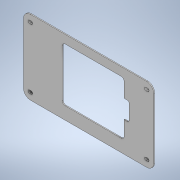
# Autodesk Inventor part: Navi base plate
Saved by Autodesk Inventor 2022 (Build 260153000, 153)
## iProperties
Created: 2021-09-22
Part Number: Navi base plate
Material: Generic
Document SubType Name: Modeling
Designer: Frank
Density: 1 g/cm^3
Appearance: Default
Author: Frank
Autodesk Inventor part; units mm, degrees
ref_plane "YZ Plane" through (0, 0, 0) normal (1, 0, 0) x (0, 1, 0)
ref_plane "XZ Plane" through (0, 0, 0) normal (0, 1, 0) x (-1, 0, 0)
ref_plane "XY Plane" through (0, 0, 0) normal (0, 0, 1) x (1, 0, 0)
sketch "Sketch1" plane through (0, 0, 0) normal (0, 0, 1) x (1, 0, 0)
  line L0 (-88.6, 55.18) -> (88.6, 55.18)
  line L1 (96.28, 47.5) -> (96.28, -47.5)
  line L2 (88.6, -55.18) -> (-88.6, -55.18)
  line L3 (-96.28, -47.5) -> (-96.28, 47.5)
  arc A0 (-96.28, -47.5) -> (-88.6, -55.18) centre (-88.6, -47.5) ccw
  arc A1 (88.6, -55.18) -> (96.28, -47.5) centre (88.6, -47.5) ccw
  arc A2 (96.28, 47.5) -> (88.6, 55.18) centre (88.6, 47.5) ccw
  arc A3 (-88.6, 55.18) -> (-96.28, 47.5) centre (-88.6, 47.5) ccw
  line L4 (85, 52.5) -> (-85, 52.5)
  line L5 (-85, 52.5) -> (-85, -52.5)
  line L6 (-85, -52.5) -> (85, -52.5)
  line L7 (85, -52.5) -> (85, 52.5)
  line L8 (85, 52.5) -> (-85, -52.5) construction
  line L9 (-85, 52.5) -> (85, -52.5) construction
  line L10 (0, -55.18) -> (0, 55.18) construction
  line L11 (-96.28, 0) -> (96.28, 0) construction
  line L12 (88.6, -47.5) -> (-88.6, -47.5) construction
  line L13 (-88.6, -47.5) -> (-88.6, 47.5) construction
  line L14 (-88.6, 47.5) -> (88.6, 47.5) construction
  line L15 (88.6, 47.5) -> (88.6, -47.5) construction
  line L16 (-92.28, -50) -> (-92.28, 50)
  line L17 (-92.28, -50) -> (-85, -50)
  line L18 (-92.28, 50) -> (-85, 50)
  line L19 (64.35, -31.825) -> (64.35, 33.825) construction
  line L20 (64.35, 33.825) -> (-61.85, 33.825) construction
  line L21 (-61.85, 33.825) -> (-61.85, -31.825) construction
  line L22 (-61.85, -31.825) -> (64.35, -31.825) construction
  line L23 (-61.85, 33.825) -> (64.35, -31.825) construction
  line L24 (-61.85, -31.825) -> (64.35, 33.825) construction
  line L25 (1.25, 0) -> (1.25, 1) construction
  line L26 (1.25, 1) -> (0, 1) construction
  line L27 (63.525, -31.825) -> (65.175, -31.825) construction
  line L28 (63.525, -30.175) -> (65.175, -30.175)
  line L29 (65.175, -33.475) -> (63.525, -33.475)
  arc A4 (63.525, -30.175) -> (63.525, -33.475) centre (63.525, -31.825) ccw
  arc A5 (65.175, -33.475) -> (65.175, -30.175) centre (65.175, -31.825) ccw
  line L30 (63.525, 33.825) -> (65.175, 33.825) construction
  line L31 (63.525, 35.475) -> (65.175, 35.475)
  line L32 (65.175, 32.175) -> (63.525, 32.175)
  arc A6 (63.525, 35.475) -> (63.525, 32.175) centre (63.525, 33.825) ccw
  arc A7 (65.175, 32.175) -> (65.175, 35.475) centre (65.175, 33.825) ccw
  line L33 (-61.025, 33.825) -> (-62.675, 33.825) construction
  line L34 (-61.025, 35.475) -> (-62.675, 35.475)
  line L35 (-62.675, 32.175) -> (-61.025, 32.175)
  arc A8 (-61.025, 32.175) -> (-61.025, 35.475) centre (-61.025, 33.825) ccw
  arc A9 (-62.675, 35.475) -> (-62.675, 32.175) centre (-62.675, 33.825) ccw
  line L36 (-61.025, -31.825) -> (-62.675, -31.825) construction
  line L37 (-61.025, -30.175) -> (-62.675, -30.175)
  line L38 (-62.675, -33.475) -> (-61.025, -33.475)
  arc A10 (-61.025, -33.475) -> (-61.025, -30.175) centre (-61.025, -31.825) ccw
  arc A11 (-62.675, -30.175) -> (-62.675, -33.475) centre (-62.675, -31.825) ccw
  line L39 (98.28, -57.18) -> (-98.28, -57.18)
  line L40 (-98.28, -57.18) -> (-98.28, 57.18)
  line L41 (-98.28, 57.18) -> (98.28, 57.18)
  line L42 (98.28, 57.18) -> (98.28, -57.18)
  line L43 (98.28, -57.18) -> (-98.28, 57.18) construction
  line L44 (-98.28, -57.18) -> (98.28, 57.18) construction
  line L45 (-69.85, 27.075) -> (-53.85, 27.075)
  line L46 (-53.85, 27.075) -> (-53.85, 40.575)
  line L47 (-53.85, 40.575) -> (-69.85, 40.575)
  line L48 (-69.85, 40.575) -> (-69.85, 27.075)
  line L49 (-69.85, 27.075) -> (-53.85, 40.575) construction
  line L50 (-53.85, 27.075) -> (-69.85, 40.575) construction
  line L51 (-53.85, -38.575) -> (-69.85, -38.575)
  line L52 (-69.85, -38.575) -> (-69.85, -25.075)
  line L53 (-69.85, -25.075) -> (-53.85, -25.075)
  line L54 (-53.85, -25.075) -> (-53.85, -38.575)
  line L55 (-53.85, -38.575) -> (-69.85, -25.075) construction
  line L56 (-69.85, -38.575) -> (-53.85, -25.075) construction
  line L57 (56.35, -38.575) -> (72.35, -38.575)
  line L58 (72.35, -38.575) -> (72.35, -25.075)
  line L59 (72.35, -25.075) -> (56.35, -25.075)
  line L60 (56.35, -25.075) -> (56.35, -38.575)
  line L61 (56.35, -38.575) -> (72.35, -25.075) construction
  line L62 (72.35, -38.575) -> (56.35, -25.075) construction
  line L63 (72.35, 40.575) -> (56.35, 40.575)
  line L64 (56.35, 40.575) -> (56.35, 27.075)
  line L65 (56.35, 27.075) -> (72.35, 27.075)
  line L66 (72.35, 27.075) -> (72.35, 40.575)
  line L67 (72.35, 40.575) -> (56.35, 27.075) construction
  line L68 (56.35, 40.575) -> (72.35, 27.075) construction
  line L69 (-22.75, -21.25) -> (35.25, -21.25) construction
  line L70 (35.25, -21.25) -> (35.25, 27.75) construction
  line L71 (35.25, 27.75) -> (-22.75, 27.75) construction
  line L72 (-22.75, 27.75) -> (-22.75, -21.25) construction
  line L73 (-22.75, -21.25) -> (35.25, 27.75) construction
  line L74 (35.25, -21.25) -> (-22.75, 27.75) construction
  line L75 (-22.75, -31.25) -> (35.25, -31.25)
  line L76 (45.25, -21.25) -> (45.25, 27.75)
  line L77 (35.25, 37.75) -> (-22.75, 37.75)
  line L78 (-32.75, 27.75) -> (-32.75, -21.25)
  line L79 (-32.75, -31.25) -> (45.25, 37.75) construction
  line L80 (45.25, -31.25) -> (-32.75, 37.75) construction
  arc A12 (-22.75, 37.75) -> (-32.75, 27.75) centre (-22.75, 27.75) ccw
  arc A13 (-32.75, -21.25) -> (-22.75, -31.25) centre (-22.75, -21.25) ccw
  arc A14 (35.25, -31.25) -> (45.25, -21.25) centre (35.25, -21.25) ccw
  arc A15 (45.25, 27.75) -> (35.25, 37.75) centre (35.25, 27.75) ccw
  line L81 (59.25, 16.75) -> (59.25, -10.25)
  line L82 (59.25, -10.25) -> (45.25, -10.25)
  line L83 (45.25, 16.75) -> (59.25, 16.75)
  line L84 (59.25, 3.25) -> (6.25, 3.25) construction
  line L85 (-17.5, -52.7) -> (-17.5, -31.25)
  line L86 (-17.5, -52.7) -> (17.5, -52.7)
  line L87 (17.5, -52.7) -> (17.5, -31.25)
  line L88 (0, 0) -> (0, -52.7) construction
  point P0 (0, 0)
  point P1 (0, 0)
  point P2 (0, -60)
  point P3 (-64.35, 17.825)
  point P4 (-64.35, 14.525)
  point P5 (61.85, 17.825)
  point P6 (61.85, 14.525)
  point P7 (61.85, 83.475)
  point P8 (61.85, 80.175)
  point P9 (-64.35, 80.175)
  point P10 (-64.35, 83.475)
  point P11 (0, -52.5)
  point P12 (0, 0)
  point P13 (0, 0)
  point P14 (-92.28, 0)
  point P15 (0, 0)
  point P16 (1.25, 1)
  point P17 (204.35, 170.6447)
  point P18 (204.35, 167.7053)
  point P19 (0, 0)
  dimension "d0" = 7.68
  dimension "d1" = 170
  dimension "d2" = 105
  dimension "d3" = 177.2
  dimension "d4" = 95
  dimension "d5" = 100
  dimension "d6" = 4
  dimension "d7" = 65.65
  dimension "d8" = 126.2
  dimension "d9" = 1.25
  dimension "d10" = 1
  dimension "d11" = 1.65
  dimension "d12" = 3.3
  dimension "d13" = 60
  dimension "d14" = 2
  dimension "d15" = 2
  dimension "d16" = 13.5
  dimension "d17" = 16
  dimension "d18" = 58
  dimension "d19" = 49
  dimension "d20" = 3.25
  dimension "d21" = 10
  dimension "d22" = 53
  dimension "d23" = 27
  dimension "d24" = 6.25
  dimension "d25" = 0.2
  dimension "d26" = 35
  constraints: 186 end point, 34 midpoint, 32 point on circle, 32 tangent, 26 parallel, 22 perpendicular, 21 point on line, 16 centre point, 11 horizontal, 9 equal length, 9 equal radius, 4 coincident, 1 vertical, 1 vertical alignment, 1 other
  measures "d0" radius of A0
  measures "d1" distance between parallel lines of L7 L5
  measures "d2" distance between parallel lines of L4 L6
  measures "d3" distance between parallel lines of L13 L15
  measures "d4" distance between parallel lines of L14 L12
  measures "d5" distance of L16.start L16.end
  measures "d6" distance between parallel lines of L3 L16
  measures "d7" distance between parallel lines of L20 L22
  measures "d8" distance between parallel lines of L21 L19
  measures "d9" distance between parallel lines of L10 L25
  measures "d10" distance between parallel lines of L11 L26
  measures "d11" distance of L27.start L27.end
  measures "d12" distance between parallel lines of L28 L29
  measures "d13" distance of point (0, -60) point (0, 0)
  measures "d14" distance between parallel lines of L41 L0
  measures "d15" distance between parallel lines of L40 L3
  measures "d16" distance of L47.end L45.start
  measures "d17" distance of L46.end L47.end
  measures "d18" distance of L70.end L71.end
  measures "d19" distance of L71.end L69.start
  measures "d20" vertical distance of L84.end point (0, 0)
  measures "d21" radius of A12
  measures "d22" distance from line of L84.end L81
  measures "d23" distance of L81.start L81.end
  measures "d24" horizontal distance of point (0, 0) L84.end
  measures "d25" distance between parallel lines of L6 L86
  measures "d26" distance between parallel lines of L87 L85
extrude "Extrusion1" add sketch "Sketch1" along normal blind 1 contours L7 L6 L87 L75 A14 L76 L82 L81 L83 A15 L77 A12 L78 A13 L85 L5 L4 | L6 L85 L75 L87 | L76 L83 L81 L82 | L48 L47 L46 L45 | L51 L52 L53 L54 | L60 L59 L58 L57 | L66 L65 L64 L63
sketch "Sketch2" plane through (0, 0, 1) normal (0, 0, 1) x (1, 0, 0)
  arc A0 (65.175, 32.175) -> (65.175, 35.475) centre (65.175, 33.825) ccw projected
  line L0 (65.175, 35.475) -> (63.525, 35.475) projected
  arc A1 (63.525, 35.475) -> (63.525, 32.175) centre (63.525, 33.825) ccw projected
  line L1 (63.525, 32.175) -> (65.175, 32.175) projected
  arc A2 (35.25, -31.25) -> (45.25, -21.25) centre (35.25, -21.25) ccw projected
  line L2 (45.25, -21.25) -> (45.25, 27.75) projected
  arc A3 (45.25, 27.75) -> (35.25, 37.75) centre (35.25, 27.75) ccw projected
  line L3 (35.25, 37.75) -> (-22.75, 37.75) projected
  arc A4 (-22.75, 37.75) -> (-32.75, 27.75) centre (-22.75, 27.75) ccw projected
  line L4 (-32.75, 27.75) -> (-32.75, -21.25) projected
  arc A5 (-32.75, -21.25) -> (-22.75, -31.25) centre (-22.75, -21.25) ccw projected
  line L5 (-22.75, -31.25) -> (35.25, -31.25) projected
  arc A6 (65.175, -33.475) -> (65.175, -30.175) centre (65.175, -31.825) ccw projected
  line L6 (65.175, -30.175) -> (63.525, -30.175) projected
  arc A7 (63.525, -30.175) -> (63.525, -33.475) centre (63.525, -31.825) ccw projected
  line L7 (63.525, -33.475) -> (65.175, -33.475) projected
  line L8 (-61.025, -30.175) -> (-62.675, -30.175) projected
  arc A8 (-62.675, -30.175) -> (-62.675, -33.475) centre (-62.675, -31.825) ccw projected
  line L9 (-62.675, -33.475) -> (-61.025, -33.475) projected
  arc A9 (-61.025, -33.475) -> (-61.025, -30.175) centre (-61.025, -31.825) ccw projected
  line L10 (-61.025, 35.475) -> (-62.675, 35.475) projected
  arc A10 (-62.675, 35.475) -> (-62.675, 32.175) centre (-62.675, 33.825) ccw projected
  line L11 (-62.675, 32.175) -> (-61.025, 32.175) projected
  arc A11 (-61.025, 32.175) -> (-61.025, 35.475) centre (-61.025, 33.825) ccw projected
  line L12 (85, -52.5) -> (-85, -52.5) projected
  line L13 (-85, -52.5) -> (-85, 52.5) projected
  line L14 (-85, 52.5) -> (85, 52.5) projected
  line L15 (85, 52.5) -> (85, -52.5) projected
  line L16 (63.525, 33.825) -> (65.175, 33.825) construction
  line L17 (-62.675, -31.825) -> (-61.025, -31.825) construction
  line L18 (64.35, -39.325) -> (-61.85, -39.325)
  line L19 (-69.35, -31.825) -> (-69.35, 33.825)
  line L20 (-61.85, 41.325) -> (64.35, 41.325)
  line L21 (71.85, 33.825) -> (71.85, -31.825)
  line L22 (71.85, -39.325) -> (-69.35, 41.325) construction
  line L23 (-69.35, -39.325) -> (71.85, 41.325) construction
  arc A12 (71.85, 33.825) -> (64.35, 41.325) centre (64.35, 33.825) ccw
  arc A13 (-61.85, 41.325) -> (-69.35, 33.825) centre (-61.85, 33.825) ccw
  arc A14 (-69.35, -31.825) -> (-61.85, -39.325) centre (-61.85, -31.825) ccw
  arc A15 (64.35, -39.325) -> (71.85, -31.825) centre (64.35, -31.825) ccw
  point P0 (0, 0)
  point P1 (1.25, 1)
  point P2 (-61.85, -31.825)
  dimension "d29" = 7.5
  constraints: 16 end point, 8 point on circle, 8 point on line, 8 tangent, 4 centre point, 4 midpoint, 3 equal radius, 3 horizontal, 2 coincident, 2 parallel, 1 perpendicular
  measures "d29" radius of A12
extrude "Extrusion2" cut sketch "Sketch2" against normal through all contours L18 A14 L19 A13 L20 A12 L21 A15 keep common part
sketch "Sketch3" plane through (0, 0, 1) normal (0, 0, 1) x (1, 0, 0)
  arc A0 (64.35, -39.325) -> (71.85, -31.825) centre (64.35, -31.825) ccw projected
  line L0 (64.35, -39.325) -> (-61.85, -39.325) projected
  arc A1 (-69.35, -31.825) -> (-61.85, -39.325) centre (-61.85, -31.825) ccw projected
  line L1 (-69.35, -31.825) -> (-69.35, 33.825) projected
  arc A2 (-61.85, 41.325) -> (-69.35, 33.825) centre (-61.85, 33.825) ccw projected
  line L2 (-61.85, 41.325) -> (64.35, 41.325) projected
  arc A3 (71.85, 33.825) -> (64.35, 41.325) centre (64.35, 33.825) ccw projected
  line L3 (71.85, 33.825) -> (71.85, -31.825) projected
  arc A4 (65.175, 32.175) -> (65.175, 35.475) centre (65.175, 33.825) ccw projected
  line L4 (65.175, 35.475) -> (63.525, 35.475) projected
  arc A5 (63.525, 35.475) -> (63.525, 32.175) centre (63.525, 33.825) ccw projected
  line L5 (63.525, 32.175) -> (65.175, 32.175) projected
  arc A6 (35.25, -31.25) -> (45.25, -21.25) centre (35.25, -21.25) ccw projected
  line L6 (45.25, -21.25) -> (45.25, 27.75) projected
  arc A7 (45.25, 27.75) -> (35.25, 37.75) centre (35.25, 27.75) ccw projected
  line L7 (35.25, 37.75) -> (-22.75, 37.75) projected
  arc A8 (-22.75, 37.75) -> (-32.75, 27.75) centre (-22.75, 27.75) ccw projected
  line L8 (-32.75, 27.75) -> (-32.75, -21.25) projected
  arc A9 (-32.75, -21.25) -> (-22.75, -31.25) centre (-22.75, -21.25) ccw projected
  line L9 (-22.75, -31.25) -> (35.25, -31.25) projected
  arc A10 (65.175, -33.475) -> (65.175, -30.175) centre (65.175, -31.825) ccw projected
  line L10 (65.175, -30.175) -> (63.525, -30.175) projected
  arc A11 (63.525, -30.175) -> (63.525, -33.475) centre (63.525, -31.825) ccw projected
  line L11 (63.525, -33.475) -> (65.175, -33.475) projected
  line L12 (-61.025, -30.175) -> (-62.675, -30.175) projected
  arc A12 (-62.675, -30.175) -> (-62.675, -33.475) centre (-62.675, -31.825) ccw projected
  line L13 (-62.675, -33.475) -> (-61.025, -33.475) projected
  arc A13 (-61.025, -33.475) -> (-61.025, -30.175) centre (-61.025, -31.825) ccw projected
  line L14 (-61.025, 35.475) -> (-62.675, 35.475) projected
  arc A14 (-62.675, 35.475) -> (-62.675, 32.175) centre (-62.675, 33.825) ccw projected
  line L15 (-62.675, 32.175) -> (-61.025, 32.175) projected
  arc A15 (-61.025, 32.175) -> (-61.025, 35.475) centre (-61.025, 33.825) ccw projected
  line L16 (-61.025, 30.975) -> (-62.675, 30.975)
  arc A16 (-62.675, 36.675) -> (-62.675, 30.975) centre (-62.675, 33.825) ccw
  line L17 (-62.675, 36.675) -> (-61.025, 36.675)
  arc A17 (-61.025, 30.975) -> (-61.025, 36.675) centre (-61.025, 33.825) ccw
  arc A18 (65.175, 30.975) -> (65.175, 36.675) centre (65.175, 33.825) ccw
  line L18 (65.175, 30.975) -> (63.525, 30.975)
  arc A19 (63.525, 36.675) -> (63.525, 30.975) centre (63.525, 33.825) ccw
  line L19 (63.525, 36.675) -> (65.175, 36.675)
  arc A20 (65.175, -34.675) -> (65.175, -28.975) centre (65.175, -31.825) ccw
  line L20 (65.175, -34.675) -> (63.525, -34.675)
  arc A21 (63.525, -28.975) -> (63.525, -34.675) centre (63.525, -31.825) ccw
  line L21 (63.525, -28.975) -> (65.175, -28.975)
  line L22 (-61.025, -28.975) -> (-62.675, -28.975)
  arc A22 (-62.675, -28.975) -> (-62.675, -34.675) centre (-62.675, -31.825) ccw
  line L23 (-62.675, -34.675) -> (-61.025, -34.675)
  arc A23 (-61.025, -34.675) -> (-61.025, -28.975) centre (-61.025, -31.825) ccw
  point P0 (0, 0)
  dimension "d32" = 5.7
  constraints: 16 end point, 16 point on circle, 8 centre point, 3 equal radius, 12 other
  measures "d32" distance of L17.start L16.end
extrude "Extrusion3" add sketch "Sketch3" against normal blind 3 contours L16 A16 L17 A17 | L18 A19 L19 A18 | L20 A21 L21 A20 | A23 L23 A22 L22
sketch "Sketch4" plane through (0, 0, 0) normal (0, 0, -1) x (-1, 0, 0)
  line L0 (-65.175, -28.975) -> (-63.525, -28.975) projected
  arc A0 (-63.525, -34.675) -> (-63.525, -28.975) centre (-63.525, -31.825) ccw projected
  line L1 (-63.525, -34.675) -> (-65.175, -34.675) projected
  arc A1 (-65.175, -28.975) -> (-65.175, -34.675) centre (-65.175, -31.825) ccw projected
  line L2 (-65.175, 36.675) -> (-63.525, 36.675) projected
  arc A2 (-63.525, 30.975) -> (-63.525, 36.675) centre (-63.525, 33.825) ccw projected
  line L3 (-63.525, 30.975) -> (-65.175, 30.975) projected
  arc A3 (-65.175, 36.675) -> (-65.175, 30.975) centre (-65.175, 33.825) ccw projected
  arc A4 (61.025, -28.975) -> (61.025, -34.675) centre (61.025, -31.825) ccw projected
  line L4 (61.025, -28.975) -> (62.675, -28.975) projected
  arc A5 (62.675, -34.675) -> (62.675, -28.975) centre (62.675, -31.825) ccw projected
  line L5 (62.675, -34.675) -> (61.025, -34.675) projected
  line L6 (61.025, 36.675) -> (62.675, 36.675) projected
  arc A6 (62.675, 30.975) -> (62.675, 36.675) centre (62.675, 33.825) ccw projected
  line L7 (62.675, 30.975) -> (61.025, 30.975) projected
  arc A7 (61.025, 36.675) -> (61.025, 30.975) centre (61.025, 33.825) ccw projected
  arc A8 (-71.85, -31.825) -> (-64.35, -39.325) centre (-64.35, -31.825) ccw projected
  line L8 (-71.85, -31.825) -> (-71.85, 33.825) projected
  arc A9 (-64.35, 41.325) -> (-71.85, 33.825) centre (-64.35, 33.825) ccw projected
  line L9 (-64.35, 41.325) -> (61.85, 41.325) projected
  arc A10 (69.35, 33.825) -> (61.85, 41.325) centre (61.85, 33.825) ccw projected
  line L10 (69.35, 33.825) -> (69.35, -31.825) projected
  arc A11 (61.85, -39.325) -> (69.35, -31.825) centre (61.85, -31.825) ccw projected
  line L11 (61.85, -39.325) -> (-64.35, -39.325) projected
  arc A12 (-65.175, 35.475) -> (-65.175, 32.175) centre (-65.175, 33.825) ccw projected
  line L12 (-65.175, 32.175) -> (-63.525, 32.175) projected
  arc A13 (-63.525, 32.175) -> (-63.525, 35.475) centre (-63.525, 33.825) ccw projected
  line L13 (-63.525, 35.475) -> (-65.175, 35.475) projected
  arc A14 (-45.25, -21.25) -> (-35.25, -31.25) centre (-35.25, -21.25) ccw projected
  line L14 (-35.25, -31.25) -> (22.75, -31.25) projected
  arc A15 (22.75, -31.25) -> (32.75, -21.25) centre (22.75, -21.25) ccw projected
  line L15 (32.75, -21.25) -> (32.75, 27.75) projected
  arc A16 (32.75, 27.75) -> (22.75, 37.75) centre (22.75, 27.75) ccw projected
  line L16 (22.75, 37.75) -> (-35.25, 37.75) projected
  arc A17 (-35.25, 37.75) -> (-45.25, 27.75) centre (-35.25, 27.75) ccw projected
  line L17 (-45.25, 27.75) -> (-45.25, -21.25) projected
  arc A18 (-65.175, -30.175) -> (-65.175, -33.475) centre (-65.175, -31.825) ccw projected
  line L18 (-65.175, -33.475) -> (-63.525, -33.475) projected
  arc A19 (-63.525, -33.475) -> (-63.525, -30.175) centre (-63.525, -31.825) ccw projected
  line L19 (-63.525, -30.175) -> (-65.175, -30.175) projected
  line L20 (62.675, -30.175) -> (61.025, -30.175) projected
  arc A20 (61.025, -30.175) -> (61.025, -33.475) centre (61.025, -31.825) ccw projected
  line L21 (61.025, -33.475) -> (62.675, -33.475) projected
  arc A21 (62.675, -33.475) -> (62.675, -30.175) centre (62.675, -31.825) ccw projected
  line L22 (62.675, 35.475) -> (61.025, 35.475) projected
  arc A22 (61.025, 35.475) -> (61.025, 32.175) centre (61.025, 33.825) ccw projected
  line L23 (61.025, 32.175) -> (62.675, 32.175) projected
  arc A23 (62.675, 32.175) -> (62.675, 35.475) centre (62.675, 33.825) ccw projected
  line L24 (24.25, -25.75) -> (-36.75, -25.75)
  line L25 (-39.75, -22.75) -> (-39.75, 29.25)
  line L26 (-36.75, 32.25) -> (24.25, 32.25)
  line L27 (27.25, 29.25) -> (27.25, -22.75)
  line L28 (27.25, -25.75) -> (-39.75, 32.25) construction
  line L29 (-39.75, -25.75) -> (27.25, 32.25) construction
  arc A24 (-36.75, 32.25) -> (-39.75, 29.25) centre (-36.75, 29.25) ccw
  arc A25 (27.25, 29.25) -> (24.25, 32.25) centre (24.25, 29.25) ccw
  arc A26 (24.25, -25.75) -> (27.25, -22.75) centre (24.25, -22.75) ccw
  arc A27 (-39.75, -22.75) -> (-36.75, -25.75) centre (-36.75, -22.75) ccw
  line L30 (22.75, -21.25) -> (-35.25, -21.25) construction
  line L31 (-35.25, -21.25) -> (-35.25, 27.75) construction
  line L32 (-35.25, 27.75) -> (22.75, 27.75) construction
  line L33 (22.75, 27.75) -> (22.75, -21.25) construction
  line L34 (22.75, -21.25) -> (-35.25, 27.75) construction
  line L35 (-35.25, -21.25) -> (22.75, 27.75) construction
  line L36 (24.25, -22.75) -> (-36.75, -22.75) construction
  line L37 (-36.75, -22.75) -> (-36.75, 29.25) construction
  line L38 (-36.75, 29.25) -> (24.25, 29.25) construction
  line L39 (24.25, 29.25) -> (24.25, -22.75) construction
  line L40 (24.25, -22.75) -> (-36.75, 29.25) construction
  line L41 (-36.75, -22.75) -> (24.25, 29.25) construction
  line L42 (-39.75, 13.25) -> (-43.25, 13.25)
  line L43 (-6.25, 3.25) -> (-45.25, 3.25) construction
  line L44 (-43.25, -6.75) -> (-39.75, -6.75)
  line L45 (-45.25, 11.25) -> (-45.25, -4.75)
  arc A28 (-43.25, 13.25) -> (-45.25, 11.25) centre (-43.25, 11.25) ccw
  arc A29 (-45.25, -4.75) -> (-43.25, -6.75) centre (-43.25, -4.75) ccw
  line L46 (-45.25, 27.75) -> (-45.25, -21.25) projected
  point P0 (0, 0)
  point P1 (-6.25, 3.25)
  point P2 (-45.25, 13.25)
  point P3 (-45.25, -6.75)
  dimension "d35" = 3
  dimension "d36" = 1.5
  dimension "d37" = 1.5
  dimension "d40" = 2
  dimension "d41" = 20
  constraints: 44 end point, 14 point on line, 12 point on circle, 12 tangent, 7 midpoint, 6 centre point, 6 parallel, 4 equal radius, 4 horizontal, 4 perpendicular, 3 coincident, 1 collinear, 1 vertical, 1 other
  measures "d35" radius of A24
  measures "d36" distance between parallel lines of L38 L32
  measures "d37" distance between parallel lines of L37 L31
  measures "d40" radius of A28
  measures "d41" distance from line of L44.start L42
extrude "Extrusion4" add sketch "Sketch4" against normal up to surface (1 mm away) contours L17 A29 L44 L25 A27 L24 A26 L27 A25 L26 A24 L42 A28 A17 L16 A16 L15 A15 L14 A14
body "Solid1"
